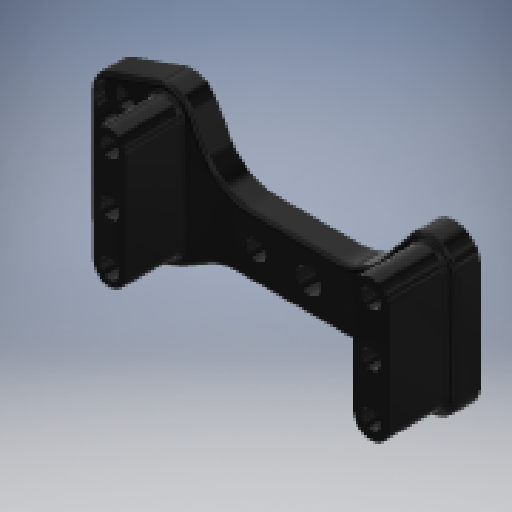
# Autodesk Inventor part: OdomPodPart2
Saved by Autodesk Inventor 2026.1 (Build 301233000, 233)
## iProperties
Created: 2025-10-06
Part Number: OdomPodPart2
Material: Plastic, Opaque Black
Document SubType Name: Modeling
Designer: Teddy
Density: 0.952 g/cm^3
Appearance: Smooth - Black
Author: Teddy
Autodesk Inventor part; units mm, degrees
ref_plane "YZ Plane" through (0, 0, 0) normal (1, 0, 0) x (0, 1, 0)
ref_plane "XZ Plane" through (0, 0, 0) normal (0, 1, 0) x (-1, 0, 0)
ref_plane "XY Plane" through (0, 0, 0) normal (0, 0, 1) x (1, 0, 0)
sketch "Sketch1" plane through (0, 0, 0) normal (0, 0, 1) x (1, 0, 0)
  circle A0 centre (-47.0732, 13.3533) radius 2.286 projected
  circle A1 centre (-47.2788, 0.1492) radius 2.286 projected
  circle A2 centre (-47.4845, -13.0592) radius 2.286 projected
  circle A3 centre (0, 0) radius 3 projected
  circle A4 centre (12.7, 0) radius 2.286
  circle A5 centre (-12.7, 0) radius 2.286
  arc A6 (12.7, -7.62) -> (12.7, 7.62) centre (12.7, 0) ccw
  line L0 (12.7, 7.62) -> (-21.6732, 7.62)
  arc A7 (-41.1289, 15.5865) -> (-53.4232, 13.3533) centre (-47.0732, 13.3533) ccw
  arc A8 (-53.4232, -13.0592) -> (-42.3761, -16.088) centre (-47.4845, -13.0592) ccw
  line L1 (-53.4232, -13.0592) -> (-53.4232, 13.3533)
  line L2 (-41.1289, 15.5865) -> (-39.6826, 11.7367)
  arc A9 (-39.6826, 11.7367) -> (-33.7382, 7.62) centre (-33.7382, 13.97) ccw construction
  line L3 (-42.3761, -16.088) -> (-39.2004, -10.7316)
  line L4 (12.7, -7.62) -> (-21.6732, -7.62)
  arc A10 (-33.7382, -7.62) -> (-39.2004, -10.7316) centre (-33.7382, -13.97) ccw construction
  arc A11 (-39.2004, -10.7316) -> (-39.0335, -10.1229) centre (-40.227, -10.1229) ccw
  arc A12 (-39.0335, 8.1635) -> (-39.6826, 11.7367) centre (-49.1935, 8.1635) ccw
  line L5 (-39.0335, 8.1635) -> (-39.0335, -10.1229)
  circle A13 centre (-59.7732, 5.026) radius 2.286 construction
  circle A14 centre (-59.7732, -7.674) radius 2.286 construction
  circle A15 centre (-59.7732, 17.726) radius 2.286 construction
  arc A16 (-57.706, 23.7301) -> (-66.1232, 17.726) centre (-59.7732, 17.726) ccw construction
  arc A17 (-66.1232, -7.674) -> (-62.1425, -13.5654) centre (-59.7732, -7.674) ccw construction
  line L6 (-57.706, 23.7301) -> (-45.006, 19.3573) construction
  line L7 (-62.1425, -13.5654) -> (-49.7003, -18.5691) construction
  line L8 (-66.1232, -7.674) -> (-66.1232, 17.726) construction
  line L9 (-59.7732, 17.726) -> (29.1268, 17.726) construction
  line L10 (29.1268, 17.726) -> (29.1268, -7.674) construction
  circle A18 centre (29.1268, 17.726) radius 2.286
  circle A19 centre (29.1268, 5.026) radius 2.286
  circle A20 centre (29.1268, -7.674) radius 2.286
  arc A21 (26.6529, -13.5223) -> (35.4768, -7.674) centre (29.1268, -7.674) ccw
  arc A22 (35.4768, 17.726) -> (24.2042, 21.7374) centre (29.1268, 17.726) ccw
  line L11 (24.2042, 21.7374) -> (12.7, 7.62)
  line L12 (35.4768, -7.674) -> (35.4768, 17.726)
  line L13 (26.6529, -13.5223) -> (12.7, -7.62)
  circle A23 centre (-34.3732, 17.726) radius 2.286
  circle A24 centre (-34.3732, 5.026) radius 2.286
  circle A25 centre (-34.3732, -7.674) radius 2.286
  arc A26 (-28.7905, 20.7518) -> (-36.4405, 23.7301) centre (-34.3732, 17.726) ccw
  line L14 (-36.4405, 23.7301) -> (-49.1405, 19.3573)
  line L15 (-28.7905, 20.7518) -> (-21.6732, 7.62)
  line L16 (-21.6732, 7.62) -> (-33.7382, 7.62) construction
  arc A27 (-32.1321, -13.6153) -> (-31.1749, -13.1597) centre (-34.3732, -7.674) ccw
  line L17 (-32.1321, -13.6153) -> (-45.3885, -18.6158)
  line L18 (-31.1749, -13.1597) -> (-21.6732, -7.62)
  line L19 (-21.6732, -7.62) -> (-33.7382, -7.62) construction
  point P0 (0, 0)
  point P1 (-39.6826, 11.7367)
  point P2 (-39.6826, 11.7367)
  dimension "d0" = 12.7
  dimension "d1" = 12.7
  dimension "d2" = 7.62
  dimension "d3" = 6.35
  dimension "d4" = 6.35
  dimension "d5" = 10.16
  dimension "d6" = 13.335
  dimension "d9" = 4.8768
  dimension "d10" = 12.7
  dimension "d11" = 12.7
  dimension "d12" = 4.572
  dimension "d13" = 6.35
  dimension "d14" = 6.35
  dimension "d15" = 6.35
  dimension "d16" = 88.9
  dimension "d17" = 12.7
  dimension "d18" = 6.35
  dimension "d25" = 63.5
  dimension "d26" = 12.7
  dimension "d27" = 12.7
  dimension "d28" = 6.35
  dimension "d29" = 12.7
  dimension "d31" = 6.35
  dimension "d32" = 12.7
  constraints: 40 end point, 30 point on circle, 29 tangent, 24 centre point, 12 coincident, 12 equal radius, 8 vertical alignment, 5 horizontal, 4 vertical, 3 horizontal alignment, 2 point on line, 1 midpoint, 1 perpendicular, 10 other
  measures "d0" distance of point (0, 0) A5.centre
  measures "d1" distance of point (0, 0) A4.centre
  measures "d2" radius of A6
  measures "d3" radius of A7
  measures "d4" radius of A9
  measures "d5" radius of A12
  measures "d6" horizontal distance of A0.centre A9.centre
  measures "d9" vertical distance of A1.centre A13.centre
  measures "d10" distance of A13.centre A15.centre
  measures "d11" distance of A13.centre A14.centre
  measures "d12" diameter of A15
  measures "d13" distance from line of L1 A14.centre
  measures "d14" radius of A16
  measures "d15" radius of A17
  measures "d16" distance of L9.start L9.end
  measures "d17" distance of A19.centre L10.end
  measures "d18" radius of A22
  measures "d25" distance of L9.end A23.centre
  measures "d26" distance of A23.centre A24.centre
  measures "d27" distance of A24.centre A25.centre
  measures "d28" radius of A26
  measures "d29" horizontal distance of A24.centre L0.end
  measures "d31" radius of A27
  measures "d32" horizontal distance of A27.centre L4.end
extrude "Extrusion1" add sketch "Sketch1" along normal blind 6.35
sketch "Sketch2" plane through (0, 0, 6.35) normal (0, 0, 1) x (1, 0, 0)
  circle A0 centre (29.1268, -7.674) radius 2.286 projected
  circle A1 centre (29.1268, 17.726) radius 2.286 projected
  line L0 (29.1268, -7.674) -> (29.1268, 17.726) construction
  line L1 (24.6818, -7.674) -> (24.6818, 17.726)
  line L2 (33.5718, 17.726) -> (33.5718, -7.674)
  arc A2 (24.6818, -7.674) -> (33.5718, -7.674) centre (29.1268, -7.674) ccw
  arc A3 (33.5718, 17.726) -> (24.6818, 17.726) centre (29.1268, 17.726) ccw
  circle A4 centre (29.1268, 5.026) radius 2.286 projected
  circle A5 centre (-34.3732, -7.674) radius 2.286 projected
  circle A6 centre (-34.3732, 5.026) radius 2.286 projected
  circle A7 centre (-34.3732, 17.726) radius 2.286 projected
  line L3 (-34.3732, -7.674) -> (-34.3732, 17.726) construction
  line L4 (-30.3383, -7.674) -> (-30.3383, 17.726)
  line L5 (-38.4081, 17.726) -> (-38.4081, -7.674)
  arc A8 (-38.4081, -7.674) -> (-30.3383, -7.674) centre (-34.3732, -7.674) ccw
  arc A9 (-30.3383, 17.726) -> (-38.4081, 17.726) centre (-34.3732, 17.726) ccw
  point P0 (0, 0)
  point P1 (29.1268, 5.026)
  dimension "d21" = 8.89
  dimension "d30" = 8.0698
  constraints: 16 end point, 8 point on circle, 8 tangent, 4 centre point, 2 midpoint, 2 parallel, 1 vertical
  measures "d21" distance between parallel lines of L2 L1
  measures "d30" distance between parallel lines of L5 L4
fillet "Fillet1" radius 12.7 4 edges at (12.7, 7.62, 3.175) (12.7, -7.62, 3.175) (-21.6732, 7.62, 3.175) (-21.6732, -7.62, 3.175)
extrude "Extrusion2" add sketch "Sketch2" along normal blind 13.97
fillet "Fillet2" radius 1.27 7 edges at (31.2556, 23.7085, 6.35) (32.6348, -12.967, 6.35) (24.6818, 5.026, 6.35) (-34.3732, -11.7089, 6.35) (-34.3732, 21.7609, 6.35) (-38.4081, 5.026, 6.35) (-30.3383, 5.026, 6.35)
sketch "Sketch3" plane through (0, 0, 6.35) normal (0, 0, 1) x (1, 0, 0)
  circle A0 centre (-47.2788, 0.1492) radius 2.286 projected
  circle A1 centre (-47.2788, 0.1492) radius 5.08
  circle A2 centre (-47.0732, 13.3533) radius 2.286 projected
  circle A3 centre (-47.0732, 13.3533) radius 5.08
  circle A4 centre (-47.4845, -13.0592) radius 2.286 projected
  circle A5 centre (-47.4845, -13.0592) radius 5.08
  point P0 (0, 0)
  dimension "d33" = 10.16
  dimension "d34" = 10.16
  dimension "d35" = 10.16
  constraints: 3 centre point, 3 coincident
  measures "d33" diameter of A1
  measures "d34" diameter of A3
  measures "d35" diameter of A5
extrude "Extrusion3" cut sketch "Sketch3" against normal blind 2.54
body "Solid1"
